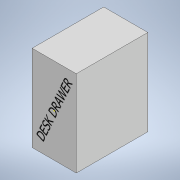
# Autodesk Inventor part: Desk Drawer
Saved by Autodesk Inventor 2020.2 (Build 242310000, 310)
## iProperties
Created: 2019-12-22
Part Number: Desk Drawer
Material: Generic
Document SubType Name: Modeling
Designer: Andrew
Density: 1 g/cm^3
Appearance: Default
d0: 27.500 in
d1: 14.125 in
d2: 22.875 in
drawer_length: 22.875 in
drawer_width: 14.125 in
drawer_height: 27.500 in
Author: Andrew
Autodesk Inventor part; units mm, degrees
ref_plane "YZ Plane" through (0, 0, 0) normal (1, 0, 0) x (0, 1, 0)
ref_plane "XZ Plane" through (0, 0, 0) normal (0, 1, 0) x (-1, 0, 0)
ref_plane "XY Plane" through (0, 0, 0) normal (0, 0, 1) x (1, 0, 0)
sketch "Sketch1" plane through (0, 0, 0) normal (0, 0, 1) x (1, 0, 0)
  line L0 (-179.3875, -349.25) -> (179.3875, -349.25)
  line L1 (179.3875, -349.25) -> (179.3875, 349.25)
  line L2 (179.3875, 349.25) -> (-179.3875, 349.25)
  line L3 (-179.3875, 349.25) -> (-179.3875, -349.25)
  line L4 (-179.3875, -349.25) -> (179.3875, 349.25) construction
  line L5 (179.3875, -349.25) -> (-179.3875, 349.25) construction
  point P0 (0, 0)
  dimension "d0" = 698.5
  dimension "d1" = 358.775
  constraints: 12 end point, 2 midpoint, 2 parallel, 1 horizontal, 1 perpendicular
  measures "d0" distance of L0.end L1.end
  measures "d1" distance of L1.end L2.end
extrude "Extrusion1" add sketch "Sketch1" against normal blind 581.025
sketch "Sketch2" plane through (0, 0, 0) normal (0, 0, 1) x (1, 0, 0)
  line L0 (-148.6954, -242.9179) -> (131.0034, 380.0218) construction
  line L1 (131.0034, 380.0218) -> (207.4732, 345.6869) construction
  line L2 (207.4732, 345.6869) -> (-72.2256, -277.2527) construction
  line L3 (-72.2256, -277.2527) -> (-148.6954, -242.9179) construction
  point P0 (0, 0)
  constraints: 2 other
equation "\"d0\" = drawer_height"
equation "\"d1\" = drawer_width"
equation "\"d2\" = drawer_length"
equation "\"drawer_length\" = 581.025"
equation "\"drawer_width\" = 358.775"
equation "\"drawer_height\" = 698.5"
body "Solid1"
